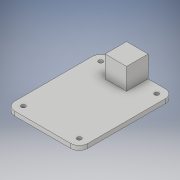
# Autodesk Inventor part: Adafruit-PowerBoost500
Saved by Autodesk Inventor 2019 (Build 230136000, 136)
## iProperties
Created: 2019-04-11
Part Number: Adafruit-PowerBoost500
Material: Generic
Document SubType Name: Modeling
Designer: Epsilon
Density: 1 g/cm^3
Appearance: Default
Author: Epsilon
Autodesk Inventor part; units mm, degrees
ref_plane "YZ Plane" through (0, 0, 0) normal (1, 0, 0) x (0, 1, 0)
ref_plane "XZ Plane" through (0, 0, 0) normal (0, 1, 0) x (-1, 0, 0)
ref_plane "XY Plane" through (0, 0, 0) normal (0, 0, 1) x (1, 0, 0)
sketch "Sketch1" plane through (0, 0, 0) normal (0, 1, 0) x (-1, 0, 0)
  line L0 (2.54, 0) -> (19.05, 0)
  line L1 (21.59, -2.54) -> (21.59, -25.4)
  line L2 (19.05, -27.94) -> (2.54, -27.94)
  line L3 (0, -25.4) -> (0, -2.54)
  arc A0 (21.59, -2.54) -> (19.05, 0) centre (19.05, -2.54) ccw
  arc A1 (2.54, 0) -> (0, -2.54) centre (2.54, -2.54) ccw
  arc A2 (0, -25.4) -> (2.54, -27.94) centre (2.54, -25.4) ccw
  arc A3 (19.05, -27.94) -> (21.59, -25.4) centre (19.05, -25.4) ccw
  circle A4 centre (19.05, -2.54) radius 0.635
  circle A5 centre (2.54, -2.54) radius 0.635
  circle A6 centre (2.54, -25.4) radius 0.635
  circle A7 centre (19.05, -25.4) radius 0.635
  point P0 (0, 0)
  point P1 (21.59, -27.94)
  point P2 (21.59, 0)
  point P3 (0, -27.94)
  dimension "d0" = 21.59
  dimension "d1" = 27.94
  dimension "d2" = 2.54
  dimension "d3" = 1.27
  dimension "d4" = 1.27
  dimension "d5" = 1.27
  dimension "d6" = 1.27
  constraints: 8 centre point, 8 end point, 8 point on circle, 8 point on line, 8 tangent, 4 coincident, 3 equal radius, 2 parallel, 1 horizontal, 1 perpendicular
  measures "d0" distance of point (21.59, -27.94) point (0, -27.94)
  measures "d1" distance of point (21.59, 0) point (21.59, -27.94)
  measures "d2" radius of A0
  measures "d3" diameter of A4
  measures "d4" diameter of A5
  measures "d5" diameter of A6
  measures "d6" diameter of A7
extrude "Extrusion1" add sketch "Sketch1" along normal blind 1.27
sketch "Sketch2" plane through (0, 1.27, 0) normal (0, 1, 0) x (1, 0, 0)
  line L0 (-19.05, 0) -> (-2.54, 0) construction
  line L1 (-10.795, 0) -> (-10.795, 27.94) construction
  line L2 (-2.54, 27.94) -> (-19.05, 27.94) construction
  line L3 (-13.97, 27.94) -> (-7.62, 27.94) construction
  line L4 (-7.62, 27.94) -> (-7.62, 21.59) construction
  line L5 (-7.62, 21.59) -> (-13.97, 21.59) construction
  line L6 (-13.97, 21.59) -> (-13.97, 27.94) construction
  line L7 (-13.97, 21.59) -> (-7.62, 21.59) construction
  line L8 (-7.62, 21.59) -> (-7.62, 27.94) construction
  line L9 (-7.62, 27.94) -> (-13.97, 27.94) construction
  line L10 (-13.97, 27.94) -> (-13.97, 21.59) construction
  line L11 (-13.97, 21.59) -> (-7.62, 21.59)
  line L12 (-7.62, 21.59) -> (-7.62, 27.94)
  line L13 (-7.62, 27.94) -> (-13.97, 27.94)
  line L14 (-13.97, 27.94) -> (-13.97, 21.59)
  point P0 (0, 0)
  dimension "d9" = 6.35
  dimension "d10" = 6.35
  dimension "d11" = 3.175
  constraints: 26 end point, 6 parallel, 3 horizontal, 3 perpendicular, 2 midpoint, 1 point on line
  measures "d9" distance between parallel lines of L4 L6
  measures "d10" distance between parallel lines of L2 L5
  measures "d11" distance between parallel lines of L1 L6
extrude "Extrusion2" add sketch "Sketch2" along normal blind 6.35
equation "\"d4\" = d3"
equation "\"d5\" = d3"
equation "\"d6\" = d3"
equation "\"d11\" = 0.5 * d10"
body "Solid1"
